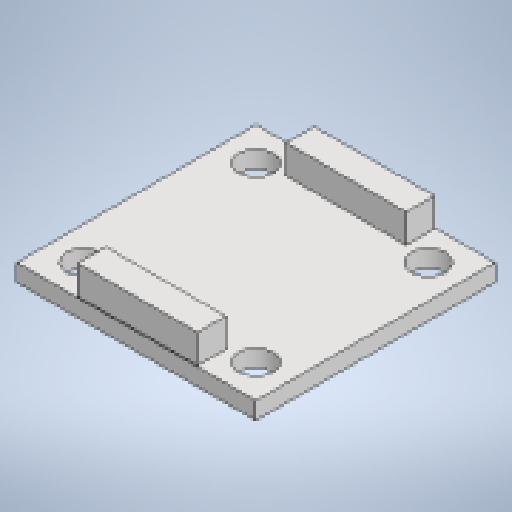
# Autodesk Inventor part: H3LIS331DL
Saved by Autodesk Inventor 2023.4 (Build 274418000, 418)
## iProperties
Created: 2024-06-07
Part Number: H3LIS331DL
Material: Generic
Document SubType Name: Modeling
Designer: Nathan Cai
Density: 1 g/cm^3
Appearance: Default
Author: Nathan Cai
Autodesk Inventor part; units mm, degrees
ref_plane "YZ Plane" through (0, 0, 0) normal (1, 0, 0) x (0, 1, 0)
ref_plane "XZ Plane" through (0, 0, 0) normal (0, 1, 0) x (-1, 0, 0)
ref_plane "XY Plane" through (0, 0, 0) normal (0, 0, 1) x (1, 0, 0)
sketch "Sketch1" plane through (0, 0, 0) normal (0, 1, 0) x (-1, 0, 0)
  line L0 (10.4, 10.4) -> (-10.4, 10.4)
  line L1 (-10.4, 10.4) -> (-10.4, -10.4)
  line L2 (-10.4, -10.4) -> (10.4, -10.4)
  line L3 (10.4, -10.4) -> (10.4, 10.4)
  line L4 (10.4, 10.4) -> (-10.4, -10.4) construction
  line L5 (-10.4, 10.4) -> (10.4, -10.4) construction
  line L6 (7.5, 7.5) -> (-7.5, 7.5) construction
  line L7 (-7.5, 7.5) -> (-7.5, -7.5) construction
  line L8 (-7.5, -7.5) -> (7.5, -7.5) construction
  line L9 (7.5, -7.5) -> (7.5, 7.5) construction
  line L10 (7.5, 7.5) -> (-7.5, -7.5) construction
  line L11 (-7.5, 7.5) -> (7.5, -7.5) construction
  circle A0 centre (7.5, -7.5) radius 1.5
  circle A1 centre (-7.5, -7.5) radius 1.5
  circle A2 centre (7.5, 7.5) radius 1.5
  circle A3 centre (-7.5, 7.5) radius 1.5
  point P0 (0, 0)
  dimension "d0" = 20.8
  dimension "d1" = 20.8
  dimension "d2" = 15
  dimension "d3" = 15
  dimension "d4" = 3
  dimension "d7" = 15
  dimension "d10" = 15
  constraints: 24 end point, 4 centre point, 4 midpoint, 4 parallel, 3 horizontal, 2 perpendicular, 1 coincident, 1 vertical, 6 other
  measures "d0" distance of L2.end L1.end
  measures "d1" distance of L1.end L0.end
  measures "d2" distance of L8.end L7.end
  measures "d3" distance of L7.end L6.end
  measures "d4" diameter of A0
  measures "d7" distance of A0.centre A1.centre
  measures "d10" distance of A0.centre A2.centre
extrude "Extrusion1" add sketch "Sketch1" along normal blind 1.5
sketch "Sketch2" plane through (0, 1.5, 0) normal (0, 1, 0) x (1, 0, 0)
  line L0 (10.4, 10.4) -> (-10.4, 10.4) projected
  line L1 (0, 10.4) -> (0, -10.4) construction
  line L2 (-10.4, -10.4) -> (10.4, -10.4) projected
  line L3 (-5.22, 10.3) -> (5.22, 10.3)
  line L4 (5.22, 10.3) -> (5.22, 7.85)
  line L5 (5.22, 7.85) -> (-5.22, 7.85)
  line L6 (-5.22, 7.85) -> (-5.22, 10.3)
  line L7 (-5.22, 10.3) -> (5.22, 7.85) construction
  line L8 (5.22, 10.3) -> (-5.22, 7.85) construction
  line L9 (-10.4, 10.4) -> (-10.4, -10.4) projected
  line L10 (-10.4, 0) -> (10.4, 0) construction
  line L11 (10.4, -10.4) -> (10.4, 10.4) projected
  line L12 (-5.22, -10.3) -> (5.22, -10.3)
  line L13 (5.22, -10.3) -> (5.22, -7.85)
  line L14 (5.22, -7.85) -> (-5.22, -7.85)
  line L15 (-5.22, -7.85) -> (-5.22, -10.3)
  line L16 (-5.22, -10.3) -> (5.22, -7.85) construction
  line L17 (5.22, -10.3) -> (-5.22, -7.85) construction
  point P0 (0, 0)
  point P1 (0, 9.075)
  point P2 (0, -9.075)
  dimension "d15" = 10.44
  dimension "d16" = 2.45
  dimension "d17" = 0.1
  constraints: 28 end point, 6 midpoint, 5 symmetric about line, 2 parallel, 1 horizontal, 1 perpendicular, 1 point on line
  measures "d15" distance of L4.end L5.end
  measures "d16" distance of L3.end L4.end
  measures "d17" distance between parallel lines of L0 L3
extrude "Extrusion2" add sketch "Sketch2" along normal blind 2.5 contours L3 L4 L5 L6 | L15 L14 L13 L12
equation "\"d7\" = d2"
equation "\"d10\" = d2"
body "Solid1"
